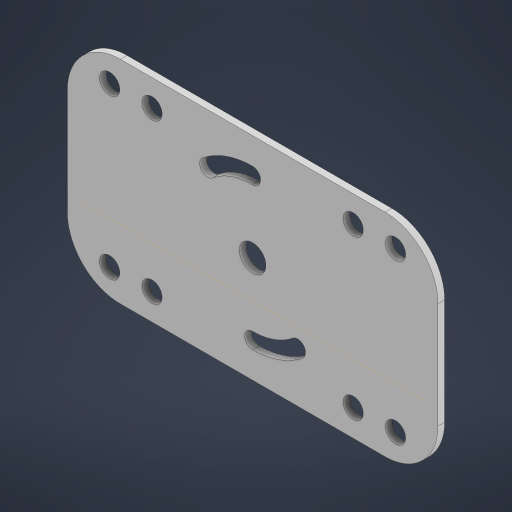
# Autodesk Inventor part: Plate
Saved by Autodesk Inventor 2024 (Build 280153000, 153)
## iProperties
Created: 2023-12-04
Part Number: Plate
Material: Generic
Document SubType Name: Modeling
Designer: calvi
Density: 1 g/cm^3
Appearance: Default
Author: calvi
Autodesk Inventor part; units mm, degrees
ref_plane "YZ Plane" through (0, 0, 0) normal (1, 0, 0) x (0, 1, 0)
ref_plane "XZ Plane" through (0, 0, 0) normal (0, 1, 0) x (-1, 0, 0)
ref_plane "XY Plane" through (0, 0, 0) normal (0, 0, 1) x (1, 0, 0)
sketch "Sketch1" plane through (0, 0, 0) normal (0, 0, 1) x (1, 0, 0)
  line L0 (-74.9559, 32.3461) -> (77.4441, 32.3461)
  line L1 (77.4441, 32.3461) -> (77.4441, -43.8539)
  line L2 (77.4441, -43.8539) -> (-74.9559, -43.8539)
  line L3 (-74.9559, -43.8539) -> (-74.9559, 32.3461)
  point P0 (0, 0)
  point P1 (77.4441, -5.7539)
  dimension "d1" = 152.4
  dimension "d2" = 76.2
  constraints: 8 end point, 2 parallel, 1 horizontal, 1 midpoint, 1 perpendicular
  measures "d1" distance between parallel lines of L1 L3
  measures "d2" distance between parallel lines of L2 L0
extrude "Extrusion1" add sketch "Sketch1" along normal blind 12.7
sketch "Sketch3" plane through (-74.9559, 32.3461, 0) normal (0, 1, 0) x (1, 0, 0)
  line L0 (0, -12.7) -> (152.4, -12.7) projected
  line L1 (152.4, 0) -> (152.4, -12.7) projected
  line L2 (0, -12.7) -> (152.4, -12.7)
  line L3 (152.4, -12.7) -> (152.4, 0)
  line L4 (152.4, 0) -> (0, 0)
  line L5 (0, 0) -> (0, -12.7)
  point P0 (74.9559, 0)
  constraints: 8 end point, 2 parallel, 1 horizontal, 1 perpendicular
extrude "Extrusion2" add sketch "Sketch3" along normal blind 12.7
sketch "Sketch5" plane through (0, 0, 12.7) normal (0, 0, 1) x (1, 0, 0)
  line L0 (1.2441, 0.5961) -> (-33.0459, 0.5961) construction
  line L1 (1.2441, 0.5961) -> (1.2441, 34.8861) construction
  line L2 (-74.9559, -43.8539) -> (77.4441, -43.8539) projected
  line L3 (77.4441, -43.8539) -> (77.4441, 45.0461) projected
  circle A0 centre (1.2441, 34.8861) radius 3.81
  line L4 (1.2441, 0.5961) -> (-29.2359, 0.5961) construction
  line L5 (1.2441, 0.5961) -> (-36.8559, 0.5961) construction
  line L6 (1.2441, 0.5961) -> (1.2441, 38.6961) construction
  line L7 (1.2441, 0.5961) -> (1.2441, 34.8861) construction
  arc A1 (1.2441, 34.8861) -> (-20.3353, 27.2445) centre (1.2441, 0.5961) ccw
  line L8 (1.2441, 0.5961) -> (-20.3353, 27.2445) construction
  line L9 (1.2441, 0.5961) -> (1.2441, 34.8861) construction
  arc A2 (1.2441, 31.0761) -> (-17.9376, 24.2835) centre (1.2441, 0.5961) ccw
  line L10 (1.2441, 0.5961) -> (-17.9376, 24.2835) construction
  line L11 (1.2441, 0.5961) -> (1.2441, 31.0761) construction
  arc A3 (1.2441, 38.6961) -> (-22.733, 30.2054) centre (1.2441, 0.5961) ccw
  line L12 (1.2441, 0.5961) -> (-22.733, 30.2054) construction
  line L13 (1.2441, 0.5961) -> (1.2441, 38.6961) construction
  circle A4 centre (-20.3353, 27.2445) radius 3.81
  circle A5 centre (1.2441, -33.6939) radius 3.81
  arc A6 (1.2441, -29.8839) -> (20.4258, -23.0913) centre (1.2441, 0.5961) ccw
  arc A7 (1.2441, -33.6939) -> (22.8235, -26.0522) centre (1.2441, 0.5961) ccw
  arc A8 (1.2441, -37.5039) -> (25.2212, -29.0131) centre (1.2441, 0.5961) ccw
  circle A9 centre (22.8235, -26.0522) radius 3.81
  line L14 (1.2441, 0.5961) -> (1.2441, -37.5039) construction
  line L15 (1.2441, 0.5961) -> (1.2441, -37.5039) construction
  line L16 (1.2441, 0.5961) -> (1.2441, -33.6939) construction
  line L17 (1.2441, 0.5961) -> (1.2441, -33.6939) construction
  line L18 (1.2441, 0.5961) -> (1.2441, -33.6939) construction
  line L19 (1.2441, 0.5961) -> (1.2441, -29.8839) construction
  line L20 (1.2441, 0.5961) -> (25.2212, -29.0131) construction
  line L21 (1.2441, 0.5961) -> (22.8235, -26.0522) construction
  line L22 (1.2441, 0.5961) -> (20.4258, -23.0913) construction
  line L23 (1.2441, 0.5961) -> (39.3441, 0.5961) construction
  line L24 (1.2441, 0.5961) -> (35.5341, 0.5961) construction
  line L25 (1.2441, 0.5961) -> (31.7241, 0.5961) construction
  point P0 (0, 0)
  point P1 (2.4882, 1.1922)
  point P2 (20.4258, -23.0913)
  dimension "d39" = 7.62
  dimension "d86" = 44.45
  dimension "d87" = 76.2
  dimension "d91" = 34.29
  dimension "d103" = 39
  dimension "d104" = 39
  dimension "d105" = 39
  dimension "d106" = 30.48
  dimension "d107" = 7.62
  dimension "d108" = 30.48
  dimension "d111" = 360
  constraints: 48 end point, 16 coincident, 16 point on circle, 8 centre point, 4 point on line, 79 other
  measures "d39" diameter of A0
  measures "d86" distance between parallel lines of L2 L0
  measures "d87" distance between parallel lines of L3 L1
  measures "d91" distance of L0.start L1.end
  measures "d103" angle of L9 L8
  measures "d104" angle of L11 L10
  measures "d105" angle of L13 L12
  measures "d106" radius of A2
  measures "d107" radial gap between concentric circles of A3 A2
  measures "d108" distance of L0.start L11.end
extrude "Extrusion4" cut sketch "Sketch5" against normal blind 57.15
sketch "Sketch7" plane through (0, 0, 12.7) normal (0, 0, 1) x (1, 0, 0)
  line L0 (-74.9559, -43.8539) -> (-74.9559, 45.0461) projected
  line L1 (-74.9559, 45.0461) -> (1.2441, 45.0461)
  line L2 (1.2441, 45.0461) -> (1.2441, 0.5961)
  line L3 (1.2441, 0.5961) -> (-74.9559, 0.5961)
  line L4 (-74.9559, 0.5961) -> (-74.9559, 45.0461)
  line L5 (77.4441, -43.8539) -> (77.4441, 45.0461) projected
  line L6 (-74.9559, -43.8539) -> (77.4441, -43.8539) projected
  point P0 (0, 0)
  dimension "d52" = 76.2
  dimension "d63" = 44.45
  constraints: 8 end point, 2 parallel, 1 horizontal, 1 perpendicular
  measures "d52" distance between parallel lines of L5 L2
  measures "d63" distance between parallel lines of L6 L3
sketch "Sketch8" plane through (0, 0, 12.7) normal (0, 0, 1) x (1, 0, 0)
  circle A0 centre (1.2441, 0.5961) radius 6.35
  line L0 (77.4441, -43.8539) -> (77.4441, 45.0461) projected
  line L1 (-74.9559, -43.8539) -> (77.4441, -43.8539) projected
  point P0 (0, 0)
  point P1 (77.4441, -18.4539)
  point P2 (77.4441, 19.6461)
  dimension "d55" = 12.7
  dimension "d56" = 76.2
  dimension "d57" = 44.45
  constraints: 1 centre point
  measures "d55" diameter of A0
  measures "d56" distance from line of L0 A0.centre
  measures "d57" distance from line of L1 A0.centre
extrude "Extrusion6" cut sketch "Sketch8" against normal blind 42.8625
sketch "Sketch11" plane through (0, 0, 0) normal (0, 0, -1) x (-1, 0, 0)
  line L0 (-77.4441, -43.8539) -> (-77.4441, 45.0461) projected
  line L1 (74.9559, -43.8539) -> (-77.4441, -43.8539) projected
  line L2 (-77.4441, 45.0461) -> (74.9559, 45.0461)
  line L3 (74.9559, 45.0461) -> (74.9559, -43.8539)
  line L4 (74.9559, -43.8539) -> (-77.4441, -43.8539)
  line L5 (-77.4441, -43.8539) -> (-77.4441, 45.0461)
  point P0 (0, 0)
  constraints: 8 end point, 2 parallel, 1 horizontal, 1 perpendicular
extrude "Extrusion8" cut sketch "Sketch11" against normal blind 9.525
ref_plane "Work Plane1" through (-74.9559, -17.1839, 12.7) normal (0, -1, 0) x (1, 0, 0)
sketch "Sketch13" plane through (77.4441, -43.8539, 12.7) normal (1, 0, 0) x (0, 0, -1)
  line L0 (0, 0) -> (0, 88.9) projected
  line L1 (3.175, 0) -> (0, 0) projected
  line L2 (0, 88.9) -> (3.175, 88.9)
  line L3 (3.175, 88.9) -> (3.175, 0)
  line L4 (3.175, 0) -> (0, 0)
  line L5 (0, 0) -> (0, 88.9)
  point P0 (12.7, 43.8539)
  constraints: 8 end point, 2 parallel, 1 horizontal, 1 perpendicular
extrude "Extrusion10" add sketch "Sketch13" along normal blind 12.7
sketch "Sketch14" plane through (-74.9559, -43.8539, 12.7) normal (-1, 0, 0) x (0, 0, 1)
  line L0 (-3.175, 88.9) -> (-3.175, 0) projected
  line L1 (0, 0) -> (0, 88.9) projected
  line L2 (-3.175, 88.9) -> (0, 88.9)
  line L3 (0, 88.9) -> (0, 0)
  line L4 (0, 0) -> (-3.175, 0)
  line L5 (-3.175, 0) -> (-3.175, 88.9)
  point P0 (-12.7, 43.8539)
  constraints: 8 end point, 2 parallel, 1 horizontal, 1 perpendicular
extrude "Extrusion11" add sketch "Sketch14" along normal blind 12.7
sketch "Sketch15" plane through (-74.9559, 45.0461, 0) normal (0, 1, 0) x (1, 0, 0)
  line L0 (165.1, -9.525) -> (-12.7, -9.525) projected
  line L1 (165.1, -12.7) -> (-12.7, -12.7) projected
  line L2 (165.1, -9.525) -> (-12.7, -9.525)
  line L3 (-12.7, -9.525) -> (-12.7, -12.7)
  line L4 (-12.7, -12.7) -> (165.1, -12.7)
  line L5 (165.1, -12.7) -> (165.1, -9.525)
  point P0 (74.9559, 0)
  point P1 (-12.7, -9.525)
  constraints: 8 end point, 2 parallel, 1 horizontal, 1 perpendicular
extrude "Extrusion12" add sketch "Sketch15" along normal blind 6.35
sketch "Sketch16" plane through (-87.6559, -43.8539, 9.525) normal (0, -1, 0) x (1, 0, 0)
  line L0 (0, 0) -> (0, 3.175) projected
  line L1 (0, 0) -> (177.8, 0)
  line L2 (177.8, 0) -> (177.8, 3.175)
  line L3 (177.8, 3.175) -> (0, 3.175)
  line L4 (0, 3.175) -> (0, 0)
  point P0 (87.6559, -9.525)
  constraints: 8 end point, 2 parallel, 1 horizontal, 1 perpendicular
extrude "Extrusion13" add sketch "Sketch16" along normal blind 6.35
sketch "Sketch17" plane through (0, 0, 12.7) normal (0, 0, 1) x (1, 0, 0)
  arc A0 (-62.2559, 51.3961) -> (-87.6559, 25.9961) centre (-62.2559, 25.9961) ccw
  line L0 (-87.6559, 51.3961) -> (90.1441, 51.3961) projected
  line L1 (-87.6559, 51.3961) -> (-87.6559, -50.2039) projected
  arc A1 (-87.6559, -24.8039) -> (-62.2559, -50.2039) centre (-62.2559, -24.8039) ccw
  arc A2 (64.7441, -50.2039) -> (90.1441, -24.8039) centre (64.7441, -24.8039) ccw
  arc A3 (90.1441, 25.9961) -> (64.7441, 51.3961) centre (64.7441, 25.9961) ccw
  line L2 (90.1441, -50.2039) -> (-87.6559, -50.2039) projected
  line L3 (90.1441, -50.2039) -> (90.1441, 51.3961) projected
  point P0 (0, 0)
  dimension "d113" = 50.8
  dimension "d114" = 50.8
  dimension "d115" = 50.8
  dimension "d116" = 50.8
  constraints: 8 point on circle, 8 point on line, 8 tangent, 4 centre point
  measures "d113" diameter of A0
  measures "d114" diameter of A1
  measures "d115" diameter of A2
  measures "d116" diameter of A3
extrude "Extrusion14" cut sketch "Sketch17" against normal blind 25.4 contours A0 L1 L0 | L0 L3 A3 | A1 L2 L1 | L3 L2 A2
sketch "Sketch18" plane through (0, 0, 12.7) normal (0, 0, 1) x (1, 0, 0)
  line L0 (-87.6559, 25.9961) -> (-87.6559, -24.8039) projected
  line L1 (-87.6559, 0.5961) -> (90.1441, 0.5961)
  line L2 (90.1441, -24.8039) -> (90.1441, 25.9961) projected
  line L3 (64.7441, -50.2039) -> (-62.2559, -50.2039) projected
  line L4 (64.7441, 51.3961) -> (-62.2559, 51.3961) projected
  line L5 (1.2441, 51.3961) -> (1.2441, -50.2039)
  circle A0 centre (-67.3359, 38.6961) radius 6.477
  circle A1 centre (-47.0159, 38.6961) radius 6.477
  circle A2 centre (-67.3359, 38.6961) radius 4.826
  circle A3 centre (-47.0159, 38.6961) radius 4.826
  circle A4 centre (-67.3359, -37.5039) radius 6.477
  circle A5 centre (-47.0159, -37.5039) radius 6.477
  circle A6 centre (-67.3359, -37.5039) radius 4.826
  circle A7 centre (-47.0159, -37.5039) radius 4.826
  circle A8 centre (69.8241, 38.6961) radius 6.477
  circle A9 centre (49.5041, 38.6961) radius 6.477
  circle A10 centre (69.8241, 38.6961) radius 4.826
  circle A11 centre (49.5041, 38.6961) radius 4.826
  circle A12 centre (69.8241, -37.5039) radius 6.477
  circle A13 centre (69.8241, -37.5039) radius 4.826
  circle A14 centre (49.5041, -37.5039) radius 4.826
  circle A15 centre (49.5041, -37.5039) radius 6.477
  point P0 (0, 0)
  dimension "d119" = 50.8
  dimension "d120" = 88.9
  dimension "d121" = 12.954
  dimension "d122" = 12.954
  dimension "d123" = 38.1
  dimension "d124" = 20.32
  dimension "d125" = 20.32
  dimension "d126" = 9.652
  dimension "d127" = 9.652
  constraints: 16 centre point, 12 symmetric about line, 8 coincident, 4 end point, 4 midpoint, 1 horizontal, 1 horizontal alignment, 1 vertical, 12 other
  measures "d119" distance between parallel lines of L3 L1
  measures "d120" distance between parallel lines of L2 L5
  measures "d121" diameter of A0
  measures "d122" diameter of A1
  measures "d123" distance from line of L1 A0.centre
  measures "d124" distance from line of L0 A0.centre
  measures "d125" distance of A1.centre A0.centre
  measures "d126" diameter of A2
  measures "d127" diameter of A3
extrude "Extrusion15" cut sketch "Sketch18" against normal blind 25.4 contours A2 | A3 | A6 | A7 | A10 | A11 | A13 | A14
body "Solid1"
